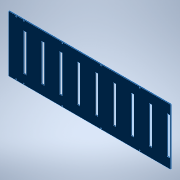
# Autodesk Inventor part: FerriteLayer
Saved by Autodesk Inventor 2021 (Build 250183000, 183)
## iProperties
Created: 2022-02-04
Part Number: FerriteLayer
Material: Generic
Document SubType Name: Modeling
Designer: tlar613
Density: 1 g/cm^3
Appearance: Default
Author: tlar613
Autodesk Inventor part; units mm, degrees
ref_plane "YZ Plane" through (0, 0, 0) normal (1, 0, 0) x (0, 1, 0)
ref_plane "XZ Plane" through (0, 0, 0) normal (0, 1, 0) x (-1, 0, 0)
ref_plane "XY Plane" through (0, 0, 0) normal (0, 0, 1) x (1, 0, 0)
sketch "Sketch1" plane through (0, 0, 0) normal (0, 0, 1) x (1, 0, 0)
  line L0 (-505, 165) -> (443.2, 165)
  line L1 (443.2, 165) -> (443.2, -165)
  line L2 (443.2, -165) -> (-505, -165)
  line L3 (-505, -165) -> (-505, 165)
  line L4 (0, 231) -> (0, -231) projected
  line L5 (-697.719, 0) -> (633.3532, 0) projected
  line L6 (3.2, 108.4) -> (18, 108.4)
  line L7 (18, 108.4) -> (18, -108.4)
  line L8 (18, -108.4) -> (3.2, -108.4)
  line L9 (3.2, -108.4) -> (3.2, 108.4)
  line L10 (-101.8, 108.4) -> (-87, 108.4)
  line L11 (-87, 108.4) -> (-87, -108.4)
  line L12 (-87, -108.4) -> (-101.8, -108.4)
  line L13 (-101.8, -108.4) -> (-101.8, 108.4)
  line L14 (-206.8, 108.4) -> (-192, 108.4)
  line L15 (-192, 108.4) -> (-192, -108.4)
  line L16 (-192, -108.4) -> (-206.8, -108.4)
  line L17 (-206.8, -108.4) -> (-206.8, 108.4)
  line L18 (-311.8, 108.4) -> (-297, 108.4)
  line L19 (-297, 108.4) -> (-297, -108.4)
  line L20 (-297, -108.4) -> (-311.8, -108.4)
  line L21 (-311.8, -108.4) -> (-311.8, 108.4)
  line L22 (-416.8, 108.4) -> (-402, 108.4)
  line L23 (-402, 108.4) -> (-402, -108.4)
  line L24 (-402, -108.4) -> (-416.8, -108.4)
  line L25 (-416.8, -108.4) -> (-416.8, 108.4)
  line L26 (108.2, 108.4) -> (123, 108.4)
  line L27 (123, 108.4) -> (123, -108.4)
  line L28 (123, -108.4) -> (108.2, -108.4)
  line L29 (108.2, -108.4) -> (108.2, 108.4)
  line L30 (213.2, 108.4) -> (228, 108.4)
  line L31 (228, 108.4) -> (228, -108.4)
  line L32 (228, -108.4) -> (213.2, -108.4)
  line L33 (213.2, -108.4) -> (213.2, 108.4)
  line L34 (318.2, 108.4) -> (333, 108.4)
  line L35 (333, 108.4) -> (333, -108.4)
  line L36 (333, -108.4) -> (318.2, -108.4)
  line L37 (318.2, -108.4) -> (318.2, 108.4)
  line L38 (438, 108.4) -> (423.2, 108.4)
  line L39 (423.2, 108.4) -> (423.2, -108.4)
  line L40 (423.2, -108.4) -> (438, -108.4)
  line L41 (438, -108.4) -> (438, 108.4)
  line L42 (-505, 159) -> (443.2, 159) construction
  line L43 (-505, -159) -> (443.2, -159) construction
  circle A0 centre (-416.1, 159) radius 3
  circle A1 centre (-190.1, 159) radius 3
  circle A2 centre (35.9, 159) radius 3
  circle A3 centre (261.9, 159) radius 3
  circle A4 centre (-460.3, 159) radius 3
  circle A5 centre (-416.1, -159) radius 3
  circle A6 centre (-190.1, -159) radius 3
  circle A7 centre (261.9, -159) radius 3
  circle A8 centre (-460.3, -159) radius 3
  circle A9 centre (35.9, -159) radius 3
  line L44 (-438.2, 153.1457) -> (-476, 153.1457)
  line L45 (-438.2, 148.8457) -> (-476, 148.8457)
  line L46 (-502.15, 126.9957) -> (-497.85, 126.9957) projected
  line L47 (-476, 153.1457) -> (-476, 148.8457) projected
  arc A10 (-476, 153.1457) -> (-502.15, 126.9957) centre (-476, 126.9957) ccw
  arc A11 (-476, 148.8457) -> (-497.85, 126.9957) centre (-476, 126.9957) ccw
  arc A12 (-469.7, 147.1564) -> (-495.85, 121.0064) centre (-469.7, 121.0064) ccw
  arc A13 (-469.7, 142.8564) -> (-491.55, 121.0064) centre (-469.7, 121.0064) ccw
  arc A14 (-463.4, 141.1671) -> (-489.55, 115.0171) centre (-463.4, 115.0171) ccw
  arc A15 (-463.4, 136.8671) -> (-485.25, 115.0171) centre (-463.4, 115.0171) ccw
  arc A16 (-457.1, 135.1778) -> (-483.25, 109.0278) centre (-457.1, 109.0278) ccw
  arc A17 (-457.1, 130.8778) -> (-478.95, 109.0278) centre (-457.1, 109.0278) ccw
  arc A18 (-450.8, 129.1885) -> (-476.95, 103.0385) centre (-450.8, 103.0385) ccw
  arc A19 (-450.8, 124.8885) -> (-472.65, 103.0385) centre (-450.8, 103.0385) ccw
  arc A20 (-444.5, 123.1992) -> (-470.65, 97.0492) centre (-444.5, 97.0492) ccw
  arc A21 (-444.5, 118.8992) -> (-466.35, 97.0492) centre (-444.5, 97.0492) ccw
  arc A22 (-438.2, 117.2099) -> (-464.35, 91.0599) centre (-438.2, 91.0599) ccw
  arc A23 (-438.2, 112.9099) -> (-460.05, 91.0599) centre (-438.2, 91.0599) ccw
  line L48 (-438.2, 123.1992) -> (-444.5, 123.1992)
  line L49 (-438.2, 118.8992) -> (-444.5, 118.8992)
  line L50 (-438.2, 124.8885) -> (-450.8, 124.8885)
  line L51 (-438.2, 129.1885) -> (-450.8, 129.1885)
  line L52 (-438.2, 130.8778) -> (-457.1, 130.8778)
  line L53 (-438.2, 135.1778) -> (-457.1, 135.1778)
  line L54 (-438.2, 141.1671) -> (-463.4, 141.1671)
  line L55 (-438.2, 136.8671) -> (-463.4, 136.8671)
  line L56 (-438.2, 142.8564) -> (-469.7, 142.8564)
  line L57 (-438.2, 147.1564) -> (-469.7, 147.1564)
  line L58 (-502.15, 126.9957) -> (-502.15, 24.9957)
  line L59 (-497.85, 126.9957) -> (-497.85, 24.9957)
  line L60 (-495.85, 121.0064) -> (-495.85, 32.3457)
  line L61 (-491.55, 121.0064) -> (-491.55, 32.3457)
  line L62 (-489.55, 115.0171) -> (-489.55, 39.6957)
  line L63 (-485.25, 115.0171) -> (-485.25, 39.6957)
  line L64 (-483.25, 109.0278) -> (-483.25, 47.0457)
  line L65 (-478.95, 109.0278) -> (-478.95, 47.0457)
  line L66 (-476.95, 103.0385) -> (-476.95, 54.3957)
  line L67 (-472.65, 103.0385) -> (-472.65, 54.3957)
  line L68 (-470.65, 97.0492) -> (-470.65, 61.7457)
  line L69 (-466.35, 97.0492) -> (-466.35, 61.7457)
  line L70 (-464.35, 91.0599) -> (-464.35, 69.0957)
  line L71 (-460.05, 91.0599) -> (-460.05, 69.0957)
  arc A24 (-460.05, 69.0957) -> (-438.2, 47.2457) centre (-438.2, 69.0957) ccw
  arc A25 (-464.35, 69.0957) -> (-438.2, 42.9457) centre (-438.2, 69.0957) ccw
  arc A26 (-466.35, 61.7457) -> (-444.5, 39.8957) centre (-444.5, 61.7457) ccw
  arc A27 (-470.65, 61.7457) -> (-444.5, 35.5957) centre (-444.5, 61.7457) ccw
  arc A28 (-476.95, 54.3957) -> (-450.8, 28.2457) centre (-450.8, 54.3957) ccw
  arc A29 (-472.65, 54.3957) -> (-450.8, 32.5457) centre (-450.8, 54.3957) ccw
  arc A30 (-478.95, 47.0457) -> (-457.1, 25.1957) centre (-457.1, 47.0457) ccw
  arc A31 (-483.25, 47.0457) -> (-457.1, 20.8957) centre (-457.1, 47.0457) ccw
  arc A32 (-485.25, 39.6957) -> (-463.4, 17.8457) centre (-463.4, 39.6957) ccw
  arc A33 (-489.55, 39.6957) -> (-463.4, 13.5457) centre (-463.4, 39.6957) ccw
  arc A34 (-491.55, 32.3457) -> (-469.7, 10.4957) centre (-469.7, 32.3457) ccw
  arc A35 (-495.85, 32.3457) -> (-469.7, 6.1957) centre (-469.7, 32.3457) ccw
  arc A36 (-497.85, 24.9957) -> (-476, 3.1457) centre (-476, 24.9957) ccw
  arc A37 (-502.15, 24.9957) -> (-476, -1.1543) centre (-476, 24.9957) ccw
  line L72 (-444.5, 39.8957) -> (-438.2, 39.8957)
  line L73 (-444.5, 35.5957) -> (-438.2, 35.5957)
  line L74 (-450.8, 32.5457) -> (-438.2, 32.5457)
  line L75 (-450.8, 28.2457) -> (-438.2, 28.2457)
  line L76 (-457.1, 25.1957) -> (-438.2, 25.1957)
  line L77 (-457.1, 20.8957) -> (-438.2, 20.8957)
  line L78 (-463.4, 17.8457) -> (-438.2, 17.8457)
  line L79 (-463.4, 13.5457) -> (-438.2, 13.5457)
  line L80 (-469.7, 10.4957) -> (-438.2, 10.4957)
  line L81 (-469.7, 6.1957) -> (-438.2, 6.1957)
  line L82 (-476, 3.1457) -> (-438.2, 3.1457)
  line L83 (-476, -1.1543) -> (-438.2, -1.1543)
  line L84 (-476, -4.2043) -> (-438.2, -4.2043)
  line L85 (-476, -8.5043) -> (-438.2, -8.5043)
  line L86 (-469.7, -11.5543) -> (-438.2, -11.5543)
  line L87 (-469.7, -15.8543) -> (-438.2, -15.8543)
  line L88 (-463.4, -18.9043) -> (-438.2, -18.9043)
  line L89 (-463.4, -23.2043) -> (-438.2, -23.2043)
  line L90 (-457.1, -26.2543) -> (-438.2, -26.2543)
  line L91 (-457.1, -30.5543) -> (-438.2, -30.5543)
  line L92 (-450.8, -33.6043) -> (-438.2, -33.6043)
  line L93 (-450.8, -37.9043) -> (-438.2, -37.9043)
  line L94 (-444.5, -40.9543) -> (-438.2, -40.9543)
  line L95 (-444.5, -45.2543) -> (-438.2, -45.2543)
  line L96 (-464.35, -87.2043) -> (-464.35, -74.4543)
  line L97 (-460.05, -87.2043) -> (-460.05, -74.4543)
  line L98 (-466.35, -93.5043) -> (-466.35, -67.1043)
  line L99 (-470.65, -93.5043) -> (-470.65, -67.1043)
  line L100 (-472.65, -99.8043) -> (-472.65, -59.7543)
  line L101 (-476.95, -99.8043) -> (-476.95, -59.7543)
  line L102 (-478.95, -106.1043) -> (-478.95, -52.4043)
  line L103 (-483.25, -106.1043) -> (-483.25, -52.4043)
  line L104 (-485.25, -112.4043) -> (-485.25, -45.0543)
  line L105 (-489.55, -112.4043) -> (-489.55, -45.0543)
  line L106 (-491.55, -118.7043) -> (-491.55, -37.7043)
  line L107 (-495.85, -118.7043) -> (-495.85, -37.7043)
  line L108 (-497.85, -125.0043) -> (-497.85, -30.3543)
  line L109 (-502.15, -125.0043) -> (-502.15, -30.3543)
  line L110 (-438.2, -115.3543) -> (-444.5, -115.3543)
  line L111 (-438.2, -119.6543) -> (-444.5, -119.6543)
  line L112 (-438.2, -121.6543) -> (-450.8, -121.6543)
  line L113 (-438.2, -125.9543) -> (-450.8, -125.9543)
  line L114 (-438.2, -127.9543) -> (-457.1, -127.9543)
  line L115 (-438.2, -132.2543) -> (-457.1, -132.2543)
  line L116 (-438.2, -134.2543) -> (-463.4, -134.2543)
  line L117 (-438.2, -138.5543) -> (-463.4, -138.5543)
  line L118 (-438.2, -140.5543) -> (-469.7, -140.5543)
  line L119 (-438.2, -144.8543) -> (-469.7, -144.8543)
  line L120 (-438.2, -146.8543) -> (-476, -146.8543)
  line L121 (-438.2, -151.1543) -> (-476, -151.1543)
  arc A38 (-438.2, -52.6043) -> (-460.05, -74.4543) centre (-438.2, -74.4543) ccw
  arc A39 (-438.2, -48.3043) -> (-464.35, -74.4543) centre (-438.2, -74.4543) ccw
  arc A40 (-444.5, -45.2543) -> (-466.35, -67.1043) centre (-444.5, -67.1043) ccw
  arc A41 (-444.5, -40.9543) -> (-470.65, -67.1043) centre (-444.5, -67.1043) ccw
  arc A42 (-450.8, -37.9043) -> (-472.65, -59.7543) centre (-450.8, -59.7543) ccw
  arc A43 (-450.8, -33.6043) -> (-476.95, -59.7543) centre (-450.8, -59.7543) ccw
  arc A44 (-457.1, -30.5543) -> (-478.95, -52.4043) centre (-457.1, -52.4043) ccw
  arc A45 (-457.1, -26.2543) -> (-483.25, -52.4043) centre (-457.1, -52.4043) ccw
  arc A46 (-463.4, -23.2043) -> (-485.25, -45.0543) centre (-463.4, -45.0543) ccw
  arc A47 (-463.4, -18.9043) -> (-489.55, -45.0543) centre (-463.4, -45.0543) ccw
  arc A48 (-469.7, -15.8543) -> (-491.55, -37.7043) centre (-469.7, -37.7043) ccw
  arc A49 (-469.7, -11.5543) -> (-495.85, -37.7043) centre (-469.7, -37.7043) ccw
  arc A50 (-476, -8.5043) -> (-497.85, -30.3543) centre (-476, -30.3543) ccw
  arc A51 (-476, -4.2043) -> (-502.15, -30.3543) centre (-476, -30.3543) ccw
  arc A52 (-460.05, -87.2043) -> (-438.2, -109.0543) centre (-438.2, -87.2043) ccw
  arc A53 (-464.35, -87.2043) -> (-438.2, -113.3543) centre (-438.2, -87.2043) ccw
  arc A54 (-466.35, -93.5043) -> (-444.5, -115.3543) centre (-444.5, -93.5043) ccw
  arc A55 (-470.65, -93.5043) -> (-444.5, -119.6543) centre (-444.5, -93.5043) ccw
  arc A56 (-472.65, -99.8043) -> (-450.8, -121.6543) centre (-450.8, -99.8043) ccw
  arc A57 (-476.95, -99.8043) -> (-450.8, -125.9543) centre (-450.8, -99.8043) ccw
  arc A58 (-478.95, -106.1043) -> (-457.1, -127.9543) centre (-457.1, -106.1043) ccw
  arc A59 (-483.25, -106.1043) -> (-457.1, -132.2543) centre (-457.1, -106.1043) ccw
  arc A60 (-485.25, -112.4043) -> (-463.4, -134.2543) centre (-463.4, -112.4043) ccw
  arc A61 (-489.55, -112.4043) -> (-463.4, -138.5543) centre (-463.4, -112.4043) ccw
  arc A62 (-491.55, -118.7043) -> (-469.7, -140.5543) centre (-469.7, -118.7043) ccw
  arc A63 (-495.85, -118.7043) -> (-469.7, -144.8543) centre (-469.7, -118.7043) ccw
  arc A64 (-497.85, -125.0043) -> (-476, -146.8543) centre (-476, -125.0043) ccw
  arc A65 (-502.15, -125.0043) -> (-476, -151.1543) centre (-476, -125.0043) ccw
  line L122 (-438.2, 32.5457) -> (-450.8, 32.5457)
  point P0 (0, 0)
  dimension "d1" = 330
  dimension "d2" = 216.8
  dimension "d3" = 14.8
  dimension "d5" = 14.8
  dimension "d8" = 14.8
  dimension "d9" = 14.8
  dimension "d11" = 14.8
  dimension "d14" = 14.8
  dimension "d16" = 14.8
  dimension "d18" = 14.8
  dimension "d20" = 438
  dimension "d21" = 14.8
  dimension "d24" = 105
  dimension "d25" = 105
  dimension "d26" = 105
  dimension "d27" = 105
  dimension "d28" = 105
  dimension "d29" = 105
  dimension "d30" = 105
  dimension "d31" = 105
  dimension "d32" = 505
  dimension "d33" = 5.2
  dimension "d34" = 6
  dimension "d35" = 6
  dimension "d36" = 6
  dimension "d37" = 88.9
  dimension "d38" = 88.9
  dimension "d39" = 226
  dimension "d40" = 226
  dimension "d41" = 226
  dimension "d42" = 226
  dimension "d43" = 226
  dimension "d44" = 226
  dimension "d45" = 44.7
  dimension "d46" = 44.7
  constraints: 238 end point, 113 point on circle, 66 centre point, 60 horizontal, 28 vertical, 20 parallel, 15 collinear, 14 point on line, 11 perpendicular, 9 equal radius, 245 other
  measures "d1" distance of L0.end L1.end
  measures "d2" distance of L6.end L7.end
  measures "d3" distance of L6.start L6.end
  measures "d5" distance of L11.end L12.end
  measures "d8" distance of L15.end L16.end
  measures "d9" distance of L19.end L20.end
  measures "d11" distance of L23.end L24.end
  measures "d14" distance of L27.end L28.end
  measures "d16" distance of L31.end L32.end
  measures "d18" distance of L35.end L36.end
  measures "d20" distance between parallel lines of L4 L41
  measures "d21" distance of L39.end L40.end
  measures "d24" distance between parallel lines of L39 L37
  measures "d25" distance between parallel lines of L37 L33
  measures "d26" distance between parallel lines of L33 L29
  measures "d27" distance between parallel lines of L29 L9
  measures "d28" distance between parallel lines of L9 L13
  measures "d29" distance between parallel lines of L13 L17
  measures "d30" distance between parallel lines of L17 L21
  measures "d31" distance between parallel lines of L21 L25
  measures "d32" distance between parallel lines of L3 L4
  measures "d33" distance between parallel lines of L1 L41
  measures "d34" distance between parallel lines of L0 L42
  measures "d35" distance between parallel lines of L2 L43
  measures "d36" diameter of A5
  measures "d37" distance from line of L3 A5.centre
  measures "d38" distance from line of A0.centre L3
  measures "d39" distance of A1.centre A0.centre
  measures "d40" distance of A2.centre A1.centre
  measures "d41" distance of A3.centre A2.centre
  measures "d42" distance of A6.centre A5.centre
  measures "d43" distance of A9.centre A6.centre
  measures "d44" distance of A7.centre A9.centre
  measures "d45" distance from line of L3 A4.centre
  measures "d46" distance from line of L3 A8.centre
extrude "Extrusion1" add sketch "Sketch1" along normal blind 5 contours L0 L4 L5 L11 L10 L13 L15 L14 L17 L19 L18 L21 L23 L22 L25 L3 | L0 L1 L5 L41 L38 L39 L35 L34 L37 L31 L30 L33 L27 L26 L29 L7 L6 L9 L4 | L5 L25 L24 L23 L21 L20 L19 L17 L16 L15 L13 L12 L11 L4 L2 L3 | L5 L9 L8 L7 L29 L28 L27 L33 L32 L31 L37 L36 L35 L39 L40 L41 L1 L2 L4 | A10 L47 A11 L46
body "Solid1"
